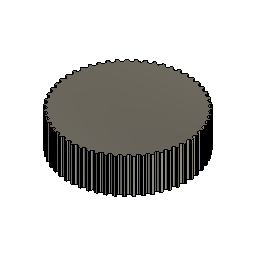
gear_55z (Autodesk Fusion 360 design; units mm, degrees)
Autodesk Fusion 360 part; units mm, degrees
sketch "Sketch1" plane through (0, 0, 0) normal (0, 0, 1) x (1, 0, 0) in component "gt2 pulley"
  circle A0 centre (0, 0) radius 17.507 construction
  circle A1 centre (0, 0) radius 16.503 construction
  line L0 (0, 0) -> (0, 17.507) construction
  line L1 (0, 0) -> (0.9995, 17.4785) construction
  line L2 (0, 0) -> (1.4067, 17.4504) construction
  circle A2 centre (0, 0) radius 17.253 construction
  arc A3 (0.3898, 17.1139) -> (0.4594, 16.8219) centre (1.3863, 17.1973) ccw
  circle A4 centre (0, 0) radius 17.103 construction
  arc A5 (0.2423, 17.2513) -> (0, 17.253) centre (0, 0) ccw
  arc A6 (0.3898, 17.1139) -> (0.2423, 17.2513) centre (0.2403, 17.1014) ccw
  arc A7 (0.4594, 16.8219) -> (0.9421, 16.4761) centre (0.9738, 17.0302) ccw
  arc A8 (0, 17.253) -> (-0.2423, 17.2513) centre (0, 0) ccw
  arc A9 (-0.2423, 17.2513) -> (-0.3898, 17.1139) centre (-0.2403, 17.1014) ccw
  arc A10 (-0.4594, 16.8219) -> (-0.3898, 17.1139) centre (-1.3863, 17.1973) ccw
  arc A11 (-0.9421, 16.4761) -> (-0.4594, 16.8219) centre (-0.9738, 17.0302) ccw
  arc A12 (0.9421, 16.4761) -> (-0.9421, 16.4761) centre (0, 0) ccw
  point P0 (1.3863, 17.1973)
  point P1 (0, 17.253)
  dimension "d18" = 35.0141
  dimension "d19" = 3.273
  dimension "d22" = 1.004
  dimension "d24" = 0.75
  dimension "d26" = 1
  dimension "d27" = 0.15
  dimension "d28" = 0.15
  dimension "d47" = 0.555
  dimension "d52" = 3.812
  constraint coincident A0.centre A1.centre
  constraint coincident A0 L0.end
  constraint vertical L0
  constraint coincident A0 L1.end
  constraint coincident A0 L2.end
  constraint concentric A1 A2
  constraint coincident A1 A7.end
  constraint coincident L1 A7.end
  constraint coincident A2 P0
  constraint coincident L2 P0
  constraint coincident P0 A3.centre
  constraint coincident A2 P1
  constraint coincident L0 P1
  constraint concentric A2 A4
  constraint coincident P1 A5.end
  constraint coincident A4 A6.centre
  constraint coincident A3.start A6.start
  constraint tangent A3 A6
  constraint tangent A3 A7
  constraint symmetric L0 A7.end A11.start
  constraint symmetric L0 A3.start A9.end
  constraint symmetric L0 A3.end A10.start
  constraint symmetric L0 A3 A10
  constraint symmetric L0 A5.start A8.end
  constraint symmetric L0 P1 A5.end
  constraint symmetric L0 A5 A8
  constraint symmetric L0 A6 A9
  constraint symmetric L0 A7 A11
  constraint coincident A1 A11.start
  constraint tangent A1 A7
  constraint coincident L1 A7.centre
  measures "d18" diameter of A0
  measures "d19" angle of L0 L1
  measures "d22" distance of A0 A1
  measures "d24" distance of A1 A2
  measures "d26" radius of A3
  measures "d27" distance of A2 A4
  measures "d28" radius of A6
  measures "d47" radius of A7
extrude "Extrude1" add sketch "Sketch1" along normal blind 10 makes body 1
pattern_circular "C-Pattern1" count 55 over 360 about axis through (0, 0, 1.75) along (0, 0, 1) of bodies 1 makes body 2 at (-2.6075, 16.2957, 6.6667) makes body 3 at (-3.0203, 16.2243, 3.3333) makes body 4 at (-6.2307, 15.2817, 6.6667) makes body 5 at (-7.3753, 14.7633, 6.6667) makes body 6 at (-9.0101, 13.8263, 6.6667) makes body 7 at (-9.8689, 13.227, 3.3333) makes body 8 at (-12.334, 10.9646, 6.6667) makes body 9 at (-13.5035, 9.4872, 6.6667) makes body 10 at (-13.7399, 9.1414, 3.3333) makes body 11 at (-15.0549, 6.7602, 6.6667) makes body 12 at (-15.9063, 4.3976, 6.6667) makes body 13 at (-16.1532, 3.3799, 3.3333) makes body 14 at (-16.3636, 2.1411, 3.3333) makes body 15 at (-16.4591, -1.2034, 6.6667) makes body 16 at (-16.4233, -1.6208, 3.3333) makes body 17 at (-16.1314, -3.4824, 3.3333) makes body 18 at (-15.6293, -5.2985, 3.3333) makes body 19 at (-14.2394, -8.3421, 6.6667) makes body 20 at (-13.5634, -9.4013, 6.6667) makes body 21 at (-11.9799, -11.3504, 6.6667) makes body 22 at (-10.608, -12.6421, 6.6667) makes body 23 at (-9.0977, -13.7689, 6.6667) makes body 24 at (-8.7453, -13.9954, 3.3333) makes body 25 at (-7.0929, -14.901, 3.3333) makes body 26 at (-3.9416, -16.0254, 6.6667) makes body 27 at (-3.5336, -16.1203, 3.3333) makes body 28 at (-0.8376, -16.4818, 6.6667) makes body 29 at (1.6729, -16.418, 6.6667) makes body 30 at (2.9173, -16.2432, 6.6667) makes body 31 at (4.7498, -15.8047, 6.6667) makes body 32 at (7.0929, -14.901, 6.6667) makes body 33 at (8.7453, -13.9954, 6.6667) makes body 34 at (9.0977, -13.7689, 3.3333) makes body 35 at (11.2359, -12.0874, 6.6667) makes body 36 at (12.5405, -10.7278, 6.6667) makes body 37 at (14.0231, -8.7008, 6.6667) makes body 38 at (14.2394, -8.3421, 3.3333) makes body 39 at (15.4163, -5.8897, 6.6667) makes body 40 at (16.1314, -3.4824, 6.6667) makes body 41 at (16.3496, -2.2449, 6.6667) makes body 42 at (16.499, -0.3666, 6.6667) makes body 43 at (16.3636, 2.1411, 6.6667) makes body 44 at (16.3039, 2.5558, 3.3333) makes body 45 at (15.9063, 4.3976, 3.3333) makes body 46 at (14.6924, 7.5155, 6.6667) makes body 47 at (13.7399, 9.1414, 6.6667) makes body 48 at (13.0046, 10.1603, 6.6667) makes body 49 at (12.334, 10.9646, 3.3333) makes body 50 at (10.3653, 12.8417, 6.6667) makes body 51 at (8.2968, 14.2658, 6.6667) makes body 52 at (7.932, 14.4718, 3.3333) makes body 53 at (4.8501, 15.7743, 6.6667) makes body 54 at (4.4481, 15.8923, 3.3333) makes body 55 at (2.6075, 16.2957, 3.3333)
sketch "Sketch2" plane through (0, 0, 10) normal (0, 0, 1) x (-1, 0, 0)
  arc A0 (-7.9008, -15.186) -> (-7.8291, -15.3744) centre (-7.7611, -15.2407) ccw
  arc A1 (-7.8291, -15.3744) -> (-7.3942, -15.5882) centre (0, 0) ccw
  arc A2 (-7.3942, -15.5882) -> (-7.2012, -15.5299) centre (-7.3298, -15.4528) ccw
  arc A3 (-7.0099, -15.2986) -> (-7.2012, -15.5299) centre (-6.3437, -16.0445) ccw
  arc A4 (-6.4241, -15.2013) -> (-7.0099, -15.2986) centre (-6.6402, -15.7126) ccw
  arc A5 (-8.1151, -14.37) -> (-6.4241, -15.2013) centre (0, 0) ccw
  arc A6 (-7.8344, -14.8932) -> (-8.1151, -14.37) centre (-8.388, -14.8532) ccw
  arc A7 (-7.9008, -15.186) -> (-7.8344, -14.8932) centre (-8.8318, -14.8211) ccw
  circle A8 centre (0, 0) radius 16.503
  constraint concentric A1 A8
extrude "Extrude2" add sketch "Sketch2" against normal blind 10 contours A5 A8 bodies 1 2 3 4 5 6 7 8 9 10 11 12 13 14 15 16 17 18 19 20 21 22 23 24 25 26 27 28 29 30 31 32 33 34 35 36 37 38 39 40 41 42 43 44 45 46 47 48 49 50 51 52 53 54 55
extrude "Extrude4" [suppressed] in component "gt2 pulley"
pattern_circular "C-Pattern7" [suppressed] in component "gt2 pulley"
extrude "Extrude3" [suppressed] in component "gt2 pulley"
pattern_circular "C-Pattern6" [suppressed] in component "gt2 pulley"
extrude "Extrude2'" [suppressed] in component "gt2 pulley"
pattern_circular "C-Pattern5" [suppressed] in component "gt2 pulley"
extrude "Extrude1'" [suppressed] in component "gt2 pulley"
pattern_circular "C-Pattern4" [suppressed] in component "gt2 pulley"
pattern_circular "C-Pattern3" [suppressed] in component "gt2 pulley"
pattern_circular "C-Pattern2" [suppressed] in component "gt2 pulley"
pattern_circular "C-Pattern1'" [suppressed] in component "gt2 pulley"
copy_body "Body->Comp1" [suppressed] in component "Component"
copy_body "Body->Comp2" [suppressed] in component "Component'"
copy_body "Body->Comp3" [suppressed] in component "Component''"
copy_body "Body->Comp4" [suppressed] in component "Component'''"
copy_body "Body->Comp5" [suppressed] in component "Component''''"
copy_body "Body->Comp6" [suppressed] in component "Component'''''"
copy_body "Body->Comp7" [suppressed] in component "Component''''''"
copy_body "Body->Comp8" [suppressed] in component "Component'''''''"
copy_body "Body->Comp9" [suppressed] in component "Component''''''''"
copy_body "Body->Comp10" [suppressed] in component "Component'''''''''"
copy_body "Body->Comp11" [suppressed] in component "Component''''''''''"
copy_body "Body->Comp12" [suppressed] in component "Component'''''''''''"
copy_body "Body->Comp13" [suppressed] in component "Component''''''''''''"
copy_body "Body->Comp14" [suppressed] in component "Component'''''''''''''"
copy_body "Body->Comp15" [suppressed] in component "Component''''''''''''''"
copy_body "Body->Comp16" [suppressed] in component "Component'''''''''''''''"
copy_body "Body->Comp17" [suppressed] in component "Component''''''''''''''''"
copy_body "Body->Comp18" [suppressed] in component "Component'''''''''''''''''"
copy_body "Body->Comp19" [suppressed] in component "Component''''''''''''''''''"
copy_body "Body->Comp20" [suppressed] in component "Component'''''''''''''''''''"
component "gt2 pulley" placed x (1, 0, 0) y (0, 1, 0) z (0, 0, 1) at (0, 0, 0)
equation "NumTeeth = 55" comment "min 20"
equation "ToothPitch = 2 mm"
equation "PullyDia = NumTeeth * ToothPitch / PI"
equation "ToothAng = ( ( 360 / NumTeeth ) * 1 deg )"
equation "TransOffsetAngle = ToothAng * 0.2"
equation "Sholulder_Radius = 0.15 mm"
equation "Root_Radius = 0.555 mm"
equation "TransRadius = 1 mm"
equation "ToolHeight = 0.75 mm"
equation "PLD = 0.254 mm"
equation "d18 = PullyDia"
equation "d19 = ToothAng / 2"
equation "d22 = PLD + ToolHeight"
equation "d24 = ToolHeight"
equation "d26 = TransRadius"
equation "d27 = Sholulder_Radius"
equation "d31 = NumTeeth"
equation "d33 = NumTeeth"
equation "d35 = NumTeeth"
equation "d37 = NumTeeth"
equation "d41 = NumTeeth"
equation "d45 = NumTeeth"
equation "d47 = Root_Radius"
equation "d50 = NumTeeth"
